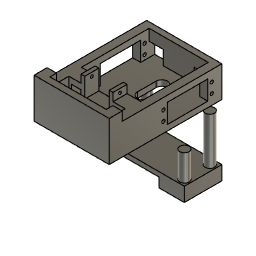
chassis_adv_LCD_mount (Autodesk Fusion 360 design; units mm, degrees)
Autodesk Fusion 360 part; units mm, degrees
sketch "Sketch1" plane through (0, 0, 0) normal (0, 0, 1) x (1, 0, 0)
  line L0 (40, -60) -> (-40, -60)
  line L1 (-40, -60) -> (-40, 60)
  line L2 (-40, 60) -> (40, 60)
  line L3 (40, 60) -> (40, -60)
  line L4 (40, -60) -> (-40, 60) construction
  line L5 (-40, -60) -> (40, 60) construction
  dimension "d1" = 80
  dimension "d2" = 120
  constraint horizontal L0
  constraint perpendicular L0 L1
  constraint parallel L0 L2
  constraint parallel L1 L3
  constraint coincident L4 origin
  constraint coincident L5 origin
  measures "d1" distance of L1.end L2.end
  measures "d2" distance of L0.end L1.end
extrude "Extrude1" add sketch "Sketch1" along normal blind 6 makes body 1
sketch "Sketch2" plane through (0, 0, 6) normal (0, 0, 1) x (-1, 0, 0)
  line L0 (-40, -60) -> (40, -60)
  line L1 (40, -60) -> (40, 60)
  line L2 (40, 60) -> (-40, 60)
  line L3 (-40, 60) -> (-40, -60)
  line L4 (40, 60) -> (-40, 60)
  line L5 (-40, 60) -> (-40, 53.15)
  line L6 (-40, 53.15) -> (40, 53.15)
  line L7 (40, 53.15) -> (40, 60)
  dimension "d5" = 6.85
  constraint horizontal L4
  constraint vertical L5
  constraint horizontal L6
  constraint vertical L7
  constraint coincident L1.end L2.start
  measures "d5" distance of L1.end L6.end
extrude "Extrude2" add sketch "Sketch2" along normal blind 36.5 contours L1 L2 L3 L4 L5 L6 L7 bodies 1
sketch "Sketch3" plane through (0, 0, 6) normal (0, 0, 1) x (-1, 0, 0)
  line L0 (40, 53.15) -> (-40, 53.15)
  line L1 (-40, 53.15) -> (-40, -60)
  line L2 (-40, -60) -> (40, -60)
  line L3 (40, -60) -> (40, 53.15)
  line L4 (40, -60) -> (31.5, -60)
  line L5 (31.5, -60) -> (31.5, -45)
  line L6 (31.5, -45) -> (40, -45)
  line L7 (40, -45) -> (40, -60)
  line L8 (40, -45) -> (31.5, -45)
  line L9 (31.5, -45) -> (31.5, -2)
  line L10 (31.5, -2) -> (40, -2)
  line L11 (40, -2) -> (40, -45)
  line L12 (40, -2) -> (31.5, -2)
  line L13 (31.5, -2) -> (31.5, 18)
  line L14 (31.5, 18) -> (40, 18)
  line L15 (40, 18) -> (40, -2)
  line L16 (0, -60) -> (0, -52.5)
  line L17 (-31.5, -60) -> (-31.5, -45)
  line L18 (-31.5, -45) -> (-40, -45)
  line L19 (-31.5, -2) -> (-40, -2)
  line L20 (-31.5, -2) -> (-31.5, 18)
  line L21 (-31.5, 18) -> (-40, 18)
  line L22 (-40, 18) -> (-40, -2)
  line L23 (-40, -45) -> (-40, -60)
  line L24 (-40, -60) -> (-31.5, -60)
  line L25 (31.5, -60) -> (-31.5, -60)
  line L26 (-31.5, -60) -> (-31.5, -54)
  line L27 (-31.5, -54) -> (31.5, -54)
  line L28 (31.5, -54) -> (31.5, -60)
  line L29 (-31.5, -45) -> (-31.5, -2)
  line L30 (-40, -2) -> (-40, -45)
  dimension "d8" = 8.5
  dimension "d9" = 15
  dimension "d10" = 8.5
  dimension "d11" = 43
  dimension "d12" = 8.5
  dimension "d13" = 20
  dimension "d14" = 63
  dimension "d15" = 6
  constraint horizontal L4
  constraint vertical L5
  constraint horizontal L6
  constraint vertical L7
  constraint coincident L2.end L3.start
  constraint horizontal L8
  constraint vertical L9
  constraint horizontal L10
  constraint vertical L11
  constraint horizontal L12
  constraint vertical L13
  constraint horizontal L14
  constraint vertical L15
  constraint midpoint L2 L16.start
  constraint perpendicular L2 L16
  constraint symmetric L2.end L16 L1.end
  constraint symmetric L4.end L16 L17.start
  constraint symmetric L5.end L16 L17.end
  constraint symmetric L6.end L16 L18.end
  constraint symmetric L9.end L16 L19.start
  constraint symmetric L10.end L16 L19.end
  constraint symmetric L13.end L16 L20.end
  constraint symmetric L14.end L16 L21.end
  constraint horizontal L25
  constraint vertical L26
  constraint horizontal L27
  constraint vertical L28
  measures "d8" distance of L2.end L4.end
  measures "d9" distance of L2.end L6.end
  measures "d10" distance of L6.end L5.end
  measures "d11" distance of L6.end L10.end
  measures "d12" distance of L10.end L9.end
  measures "d13" distance of L10.end L14.end
  measures "d14" distance of L4.end L17.start
  measures "d15" distance of L4.end L27.end
extrude "Extrude3" add sketch "Sketch3" along normal blind 20.5 contours L3 L10 L12 L13 L14 L15 | L1 L19 L20 L21 L22 | L2 L3 L4 L5 L6 L7 L8 L28 | L1 L2 L17 L18 L23 L24 L26 | L2 L5 L16 L25 L27 L28 | L2 L16 L17 L25 L26 L27 bodies 1
sketch "Sketch4" plane through (0, 60, 0) normal (0, 1, 0) x (-1, 0, 0)
  line L0 (-40, 0) -> (40, 0)
  line L1 (40, 0) -> (40, 26.5)
  line L2 (40, 26.5) -> (-40, 26.5)
  line L3 (-40, 26.5) -> (-40, 0)
  line L4 (-40, 0) -> (-31.5, 0)
  line L5 (-31.5, 0) -> (-31.5, 6)
  line L6 (-31.5, 6) -> (-40, 6)
  line L7 (-40, 6) -> (-40, 0)
  line L8 (-31.5, 6) -> (-11.5, 6)
  line L9 (-11.5, 6) -> (-11.5, 26)
  line L10 (-11.5, 26) -> (-31.5, 26)
  line L11 (-31.5, 26) -> (-31.5, 6)
  line L12 (0, 0) -> (0, 5)
  line L13 (11.5, 6) -> (11.5, 26)
  line L14 (11.5, 26) -> (31.5, 26)
  line L15 (31.5, 26) -> (31.5, 6)
  line L16 (31.5, 6) -> (11.5, 6)
  dimension "d18" = 8.5
  dimension "d19" = 6
  dimension "d20" = 20
  dimension "d21" = 20
  constraint horizontal L4
  constraint vertical L5
  constraint horizontal L6
  constraint vertical L7
  constraint coincident L0.start L3.end
  constraint horizontal L8
  constraint vertical L9
  constraint horizontal L10
  constraint vertical L11
  constraint coincident L12.start origin
  constraint perpendicular L0 L12
  constraint symmetric L5.end L12 L15.end
  constraint symmetric L8.end L12 L13.start
  constraint symmetric L9.end L12 L13.end
  constraint symmetric L10.end L12 L14.end
  measures "d18" distance of L0.start L4.end
  measures "d19" distance of L0.start L6.end
  measures "d20" distance of L5.end L8.end
  measures "d21" distance of L5.end L10.end
extrude "Extrude4" cut sketch "Sketch4" against normal blind 15 contours L8 L9 L10 L11 | L13 L14 L15 L16 bodies 1
extrude "Extrude5" add sketch "Sketch3" along normal blind 6 from surface at 20.5 contours L3 L10 L12 L13 L14 L15 | L1 L19 L20 L21 L22 | L3 L6 L8 L9 L10 L11 L12 | L1 L18 L19 L29 L30 | L2 L3 L4 L5 L6 L7 L8 L28 | L1 L2 L17 L18 L23 L24 L26 | L2 L5 L16 L25 L27 L28 | L2 L16 L17 L25 L26 L27 bodies 1
extrude "Extrude6" add 1 faces at (-11.5, 56, 12.6667) along direction (-1, 0, 0) blind 5 on bodies 1 bodies 1
extrude "Extrude7" add 1 faces at (11.5, 56, 12.6667) along direction (1, 0, 0) blind 5 on bodies 1 bodies 1
extrude "Extrude8" add 1 faces at (26.5, 56, 26) along direction (0, 0, -1) blind 5 on bodies 1 bodies 1
extrude "Extrude9" add 1 faces at (-21.5, 58, 26) along direction (0, 0, -1) blind 5 on bodies 1 bodies 1
sketch "Sketch5" plane through (0, 0, 6) normal (0, 0, 1) x (-1, 0, 0)
  line L0 (-16.5, -60) -> (-16.5, -54)
  line L1 (-16.5, -54) -> (16.5, -54)
  line L2 (16.5, -54) -> (16.5, -60)
  line L3 (16.5, -60) -> (31.5, -60)
  line L4 (31.5, -60) -> (31.5, -45)
  line L5 (31.5, -45) -> (40, -45)
  line L6 (40, -45) -> (40, -2)
  line L7 (40, -2) -> (31.5, -2)
  line L8 (31.5, -2) -> (31.5, 18)
  line L9 (31.5, 18) -> (40, 18)
  line L10 (40, 18) -> (40, 53.15)
  line L11 (40, 53.15) -> (-40, 53.15)
  line L12 (-40, 53.15) -> (-40, 18)
  line L13 (-40, 18) -> (-31.5, 18)
  line L14 (-31.5, 18) -> (-31.5, -2)
  line L15 (-31.5, -2) -> (-40, -2)
  line L16 (-40, -2) -> (-40, -45)
  line L17 (-40, -45) -> (-31.5, -45)
  line L18 (-31.5, -45) -> (-31.5, -60)
  line L19 (-31.5, -60) -> (-16.5, -60)
  line L20 (-40, 18) -> (40, 18)
  line L21 (40, 18) -> (40, 33)
  line L22 (40, 33) -> (-40, 33)
  line L23 (-40, 33) -> (-40, 18)
  line L24 (-40, 53.15) -> (-30, 53.15)
  line L25 (-30, 53.15) -> (-30, 33)
  line L26 (-30, 33) -> (-40, 33)
  line L27 (-40, 33) -> (-40, 53.15)
  line L28 (40, 53.15) -> (30, 53.15)
  line L29 (30, 53.15) -> (30, 33)
  line L30 (30, 33) -> (40, 33)
  line L31 (40, 33) -> (40, 53.15)
  dimension "d35" = 15
  dimension "d36" = 10
  dimension "d37" = 10
  constraint horizontal L20
  constraint vertical L21
  constraint horizontal L22
  constraint vertical L23
  constraint coincident L12.end L13.start
  constraint horizontal L24
  constraint vertical L25
  constraint horizontal L26
  constraint vertical L27
  constraint coincident L22 L25.end
  constraint coincident L11.end L12.start
  constraint horizontal L28
  constraint vertical L29
  constraint horizontal L30
  constraint vertical L31
  constraint coincident L22 L29.end
  constraint coincident L10.end L11.start
  measures "d35" distance of L12.end L22.end
  measures "d36" distance of L11.end L24.end
  measures "d37" distance of L10.end L28.end
extrude "Extrude10" add sketch "Sketch5" along normal blind 26.5 contours L9 L10 L12 L13 L20 L21 L22 L23 L26 L30 | L11 L12 L22 L24 L25 L26 L27 | L10 L11 L22 L28 L29 L30 L31 bodies 1
sketch "Sketch6" plane through (0, 0, 32.5) normal (0, 0, 1) x (-1, 0, 0)
  line L0 (31.5, 18) -> (31.5, -54)
  line L1 (31.5, -54) -> (-31.5, -54)
  line L2 (-31.5, -54) -> (-31.5, 18)
  line L3 (-31.5, 18) -> (31.5, 18)
  line L4 (40, -60) -> (40, 53.15)
  line L5 (40, 53.15) -> (30, 53.15)
  line L6 (30, 53.15) -> (30, 33)
  line L7 (30, 33) -> (-30, 33)
  line L8 (-30, 33) -> (-30, 53.15)
  line L9 (-30, 53.15) -> (-40, 53.15)
  line L10 (-40, 53.15) -> (-40, -60)
  line L11 (-40, -60) -> (40, -60)
  line L12 (-40, 53.15) -> (-30, 53.15)
  line L13 (-30, 53.15) -> (-30, 46.15)
  line L14 (-30, 46.15) -> (-40, 46.15)
  line L15 (-40, 46.15) -> (-40, 53.15)
  line L16 (30, 53.15) -> (40, 53.15)
  line L17 (40, 53.15) -> (40, 46.15)
  line L18 (40, 46.15) -> (30, 46.15)
  line L19 (30, 46.15) -> (30, 53.15)
  dimension "d40" = 7
  dimension "d41" = 7
  constraint horizontal L12
  constraint vertical L13
  constraint horizontal L14
  constraint vertical L15
  constraint coincident L9.end L10.start
  constraint horizontal L16
  constraint vertical L17
  constraint horizontal L18
  constraint vertical L19
  constraint coincident L5.end L6.start
  measures "d40" distance of L9.end L14.end
  measures "d41" distance of L5.end L18.end
extrude "Extrude11" add sketch "Sketch6" along normal blind 10 contours L4 L5 L6 L16 L17 L18 L19 | L8 L9 L10 L12 L13 L14 L15 bodies 1
sketch "Sketch7" plane through (0, 0, 32.5) normal (0, 0, 1) x (-1, 0, 0)
  line L0 (31.5, 18) -> (31.5, -54)
  line L1 (31.5, -54) -> (-31.5, -54)
  line L2 (-31.5, -54) -> (-31.5, 18)
  line L3 (-31.5, 18) -> (31.5, 18)
  line L4 (-30, 46.15) -> (-40, 46.15)
  line L5 (-40, 46.15) -> (-40, -60)
  line L6 (-40, -60) -> (40, -60)
  line L7 (40, -60) -> (40, 46.15)
  line L8 (40, 46.15) -> (30, 46.15)
  line L9 (30, 46.15) -> (30, 33)
  line L10 (30, 33) -> (-30, 33)
  line L11 (-30, 33) -> (-30, 46.15)
  line L12 (0, 18) -> (0, 33)
  line L13 (13, 18) -> (-13, 18)
  line L14 (-13, 18) -> (-13, 33)
  line L15 (-13, 33) -> (13, 33)
  line L16 (13, 33) -> (13, 18)
  line L17 (13, 18) -> (-13, 33) construction
  line L18 (-13, 18) -> (13, 33) construction
  line L19 (-13, 33) -> (-17, 33)
  line L20 (-17, 33) -> (-17, 18)
  line L21 (-17, 18) -> (-13, 18)
  line L22 (-13, 18) -> (-13, 33)
  line L23 (13, 33) -> (17, 33)
  line L24 (17, 33) -> (17, 18)
  line L25 (17, 18) -> (13, 18)
  line L26 (13, 18) -> (13, 33)
  point P0 (0, 25.5)
  dimension "d44" = 26
  dimension "d45" = 4
  dimension "d46" = 4
  constraint midpoint L3 L12.start
  constraint midpoint L10 L12.end
  constraint horizontal L13
  constraint perpendicular L13 L14
  constraint parallel L13 L15
  constraint parallel L14 L16
  constraint coincident L17 P0
  constraint coincident L18 P0
  constraint midpoint L12 P0
  constraint horizontal L19
  constraint vertical L20
  constraint horizontal L21
  constraint vertical L22
  constraint coincident L3 L20.end
  constraint horizontal L23
  constraint vertical L24
  constraint horizontal L25
  constraint vertical L26
  measures "d44" distance of L14.end L15.end
  measures "d45" distance of L14.end L19.end
  measures "d46" distance of L15.end L23.end
extrude "Extrude12" add sketch "Sketch7" along normal blind 9 contours L3 L10 L16 L23 L24 L25 L26 | L3 L10 L14 L19 L20 L21 L22 bodies 1
extrude "Extrude13" cut 1 faces at (4.3333, -23, 32.5) along direction (0, 0, -1) blind 12 on bodies 1 bodies 1
sketch "Sketch8" plane through (17, 0, 0) normal (1, 0, 0) x (0, 1, 0)
  line L0 (-33, 32.5) -> (-18, 32.5)
  line L1 (-18, 32.5) -> (-18, 41.5)
  line L2 (-18, 41.5) -> (-33, 41.5)
  line L3 (-33, 41.5) -> (-33, 32.5)
  line L4 (-25.5, 41.5) -> (-25.5, 37.5)
  circle A0 centre (-25.5, 37.5) radius 1.5
  dimension "d51" = 4
  dimension "d52" = 3
  constraint midpoint L2 L4.start
  constraint perpendicular L2 L4
  constraint coincident L4.end A0.centre
  measures "d51" distance of L4.start L4.end
  measures "d52" diameter of A0
extrude "Extrude14" cut sketch "Sketch8" against normal blind 40 contours A0 bodies 1
sketch "Sketch9" plane through (40, 0, 0) normal (1, 0, 0) x (0, 1, 0)
  line L0 (45, 26.5) -> (45, 6)
  line L1 (45, 6) -> (2, 6)
  line L2 (2, 6) -> (2, 26.5)
  line L3 (2, 26.5) -> (45, 26.5)
  line L4 (60, 0) -> (60, 32.5)
  line L5 (60, 32.5) -> (-46.15, 32.5)
  line L6 (-46.15, 32.5) -> (-46.15, 42.5)
  line L7 (-46.15, 42.5) -> (-60, 42.5)
  line L8 (-60, 42.5) -> (-60, 0)
  line L9 (-60, 0) -> (60, 0)
  line L10 (45, 6) -> (45, 11)
  line L11 (45, 11) -> (49.25, 11)
  circle A0 centre (49.25, 11) radius 1.75
  line L12 (45, 16.25) -> (47.125, 16.25)
  line L13 (23.5, 6) -> (23.5, 10)
  circle A1 centre (49.25, 21.5) radius 1.75
  circle A2 centre (-2.25, 11) radius 1.75
  circle A3 centre (-2.25, 21.5) radius 1.75
  dimension "d55" = 5
  dimension "d56" = 4.25
  dimension "d57" = 3.5
  constraint coincident L0.end L1.start
  constraint coincident L0 L10.end
  constraint perpendicular L10 L11
  constraint coincident L11.end A0.centre
  constraint midpoint L0 L12.start
  constraint perpendicular L0 L12
  constraint midpoint L1 L13.start
  constraint perpendicular L1 L13
  constraint symmetric A0 L12 A1
  constraint symmetric A0 L13 A2
  constraint symmetric L13 A1 A3
  measures "d55" distance of L0.end L10.end
  measures "d56" distance of L10.end L11.end
  measures "d57" diameter of A0
extrude "Extrude15" cut sketch "Sketch9" against normal blind 95 contours A0 | A1 | A2 | A3 bodies 1
sketch "Sketch10" plane through (0, 0, 6) normal (0, 0, 1) x (-1, 0, 0)
  line L0 (31.5, 18) -> (-31.5, 18)
  line L1 (-31.5, 18) -> (-31.5, -2)
  line L2 (-31.5, -2) -> (-40, -2)
  line L3 (-40, -2) -> (-40, -45)
  line L4 (-40, -45) -> (-31.5, -45)
  line L5 (-31.5, -45) -> (-31.5, -60)
  line L6 (-31.5, -60) -> (-16.5, -60)
  line L7 (-16.5, -60) -> (-16.5, -54)
  line L8 (-16.5, -54) -> (16.5, -54)
  line L9 (16.5, -54) -> (16.5, -60)
  line L10 (16.5, -60) -> (31.5, -60)
  line L11 (31.5, -60) -> (31.5, -45)
  line L12 (31.5, -45) -> (40, -45)
  line L13 (40, -45) -> (40, -2)
  line L14 (40, -2) -> (31.5, -2)
  line L15 (31.5, -2) -> (31.5, 18)
  line L16 (0, -60) -> (0, -26)
  line L17 (6, -36) -> (6, -16)
  arc A0 (6, -16) -> (-6, -16) centre (0, -16) ccw
  line L18 (-6, -16) -> (-6, -36)
  arc A1 (-6, -36) -> (6, -36) centre (0, -36) ccw
  line L19 (0, -36) -> (0, -16) construction
  point P0 (0, -26)
  dimension "d60" = 34
  dimension "d61" = 10
  dimension "d62" = 12
  constraint perpendicular L8 L16
  constraint tangent L17 A0
  constraint tangent A0 L18
  constraint parallel L17 L18
  constraint tangent L18 A1
  constraint tangent L17 A1
  constraint perpendicular L0 L19
  constraint coincident P0 L16.end
  constraint midpoint L19 P0
  measures "d60" distance of L16.start P0
  measures "d61" distance of A0.centre P0
  measures "d62" diameter of A0
extrude "Extrude16" cut sketch "Sketch10" against normal blind 20 contours L17 A0 L18 A1 bodies 1
extrude "Extrude17" add 1 faces at (-26.1667, -23, 32.5) along direction (0, 0, 1) blind 0.5 on bodies 1 bodies 1
sketch "Sketch11" plane through (0, -18, 0) normal (0, 1, 0) x (-1, 0, 0)
  line L0 (13, 41.5) -> (13, 20.5)
  line L1 (13, 20.5) -> (-13, 20.5)
  line L2 (-13, 20.5) -> (-13, 41.5)
  line L3 (-13, 41.5) -> (-17, 41.5)
  line L4 (-17, 41.5) -> (-17, 33)
  line L5 (-17, 33) -> (-31.5, 33)
  line L6 (-31.5, 33) -> (-31.5, 6)
  line L7 (-31.5, 6) -> (31.5, 6)
  line L8 (31.5, 6) -> (31.5, 33)
  line L9 (31.5, 33) -> (17, 33)
  line L10 (17, 33) -> (17, 41.5)
  line L11 (17, 41.5) -> (13, 41.5)
  line L12 (-31.5, 19.5) -> (-13, 19.5)
  line L13 (-17.25, 12) -> (-27.25, 12)
  line L14 (-27.25, 12) -> (-27.25, 27)
  line L15 (-27.25, 27) -> (-17.25, 27)
  line L16 (-17.25, 27) -> (-17.25, 12)
  line L17 (-17.25, 12) -> (-27.25, 27) construction
  line L18 (-27.25, 12) -> (-17.25, 27) construction
  line L19 (0, 20.5) -> (0, 15)
  line L20 (27.25, 12) -> (27.25, 27)
  line L21 (27.25, 27) -> (17.25, 27)
  line L22 (17.25, 27) -> (17.25, 12)
  line L23 (17.25, 12) -> (27.25, 12)
  point P0 (-22.25, 19.5)
  dimension "d67" = 10
  dimension "d68" = 15
  constraint midpoint L6 L12.start
  constraint perpendicular L2 L12
  constraint horizontal L13
  constraint perpendicular L13 L14
  constraint parallel L13 L15
  constraint parallel L14 L16
  constraint coincident L17 P0
  constraint coincident L18 P0
  constraint midpoint L12 P0
  constraint midpoint L1 L19.start
  constraint perpendicular L1 L19
  constraint symmetric L13.start L19 L22.end
  constraint symmetric L13.end L19 L20.start
  constraint symmetric L14.end L19 L20.end
  constraint symmetric L15.end L19 L21.end
  measures "d67" distance of L14.end L15.end
  measures "d68" distance of L13.end L14.end
extrude "Extrude18" cut sketch "Sketch11" against normal blind 19 contours L12 L14 L15 L16 | L12 L13 L14 L16 | L20 L21 L22 L23 bodies 1
sketch "Sketch12" plane through (0, 0, 0) normal (0, 0, -1) x (1, 0, 0)
  line L0 (-6, -36) -> (-6, -16)
  arc A0 (6, -16) -> (-6, -16) centre (0, -16) ccw
  line L1 (6, -16) -> (6, -36)
  arc A1 (-6, -36) -> (6, -36) centre (0, -36) ccw
  line L2 (-40, -60) -> (40, -60)
  line L3 (40, -60) -> (40, 60)
  line L4 (40, 60) -> (-40, 60)
  line L5 (-40, 60) -> (-40, -60)
  line L6 (-40, -60) -> (40, -60)
  line L7 (40, -60) -> (40, -20)
  line L8 (40, -20) -> (-40, -20)
  line L9 (-40, -20) -> (-40, -60)
  constraint horizontal L6
  constraint vertical L7
  constraint horizontal L8
  constraint vertical L9
  constraint coincident L3 L7.end
  constraint coincident L2.start L5.end
extrude "Extrude19" add sketch "Sketch12" along normal blind 5 from surface at 60 separate body contours L0 L1 A1 L2 L3 L5 L6 L7 L8 L9 | L0 L1 A1 L8 makes body 2
sketch "Sketch13" plane through (0, 0, -65) normal (0, 0, -1) x (1, 0, 0)
  line L0 (-40, -20) -> (-40, -60)
  line L1 (-40, -60) -> (40, -60)
  line L2 (40, -60) -> (40, -20)
  line L3 (40, -20) -> (-40, -20)
  circle A0 centre (-33.6814, -53.5328) radius 5
  circle A1 centre (33.6814, -53.5328) radius 5
  line L4 (-40, -40) -> (40, -40)
  circle A2 centre (33.6814, -26.4672) radius 5
  circle A3 centre (-33.6814, -26.4672) radius 5
  dimension "d74" = 10
  constraint midpoint L0 L4.start
  constraint midpoint L2 L4.end
  constraint symmetric A0 L4 A3
  constraint symmetric A1 L4 A2
  measures "d74" diameter of A0
extrude "Extrude20" add sketch "Sketch13" against normal blind 50 from surface at -5 contours A0 | A1 bodies 2
extrude "Extrude21" add sketch "Sketch13" against normal blind 28 from surface at -5 contours A2 bodies 2
sketch "Sketch14" plane through (0, 0, -65) normal (0, 0, -1) x (1, 0, 0)
  line L0 (-40, -20) -> (-40, -60)
  line L1 (-40, -60) -> (40, -60)
  line L2 (40, -60) -> (40, -20)
  line L3 (40, -20) -> (-40, -20)
  line L4 (40, -60) -> (-40, -60)
  line L5 (40, -20) -> (13, -20)
  line L6 (13, -20) -> (13, -48)
  line L7 (13, -48) -> (-40, -48)
  dimension "d81" = 27
  dimension "d82" = 28
  constraint coincident L1.end L2.start
  constraint coincident L0.end L1.start
  constraint coincident L2.end L3.start
  constraint perpendicular L2 L5
  constraint perpendicular L5 L6
  constraint coincident L0 L7.end
  constraint perpendicular L0 L7
  measures "d81" distance of L2.end L5.end
  measures "d82" distance of L5.end L6.end
extrude "Extrude22" add sketch "Sketch14" along normal blind 10 contours L0 L1 L2 L3 L4 L5 L6 L7 bodies 2
sketch "Sketch15" plane through (0, 0, -65) normal (0, 0, -1) x (1, 0, 0)
  line L0 (13, -48) -> (13, -20)
  line L1 (13, -20) -> (-40, -20)
  line L2 (-40, -20) -> (-40, -48)
  line L3 (-40, -48) -> (13, -48)
  line L4 (-40, -34) -> (13, -34) construction
  line L5 (-40, -34) -> (-40, -32) construction
  line L6 (-40, -34) -> (-40, -36) construction
  line L7 (-40, -32) -> (-39, -32) construction
  line L8 (-39, -32) -> (-37, -32)
  line L9 (-37, -32) -> (-37, -36)
  line L10 (-37, -36) -> (-39, -36)
  line L11 (-39, -36) -> (-39, -32)
  dimension "d85" = 2
  dimension "d86" = 2
  dimension "d87" = 2
  constraint midpoint L2 L4.start
  constraint midpoint L0 L4.end
  constraint perpendicular L4 L5
  constraint perpendicular L4 L6
  constraint perpendicular L5 L7
  constraint parallel L7 L8
  constraint perpendicular L4 L9
  constraint perpendicular L9 L10
  constraint perpendicular L7 L11
  measures "d85" distance of L4.start L5.end
  measures "d86" distance of L4.start L6.end
  measures "d87" distance of L7.end L8.end
extrude "Extrude23" cut sketch "Sketch15" against normal blind 19 contours L8 L9 L10 L11 bodies 2
